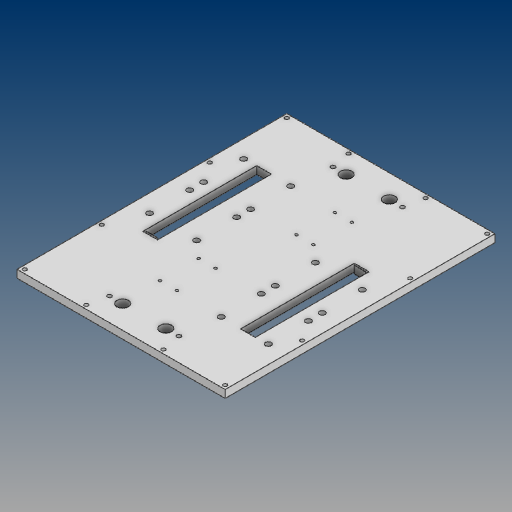
# Autodesk Inventor part: 06_Tam_de_01
Saved by Autodesk Inventor 2021 (Build 250183000, 183)
## iProperties
Created: 2024-03-25
Part Number: 06_Tam_de_01
Material: Generic
Document SubType Name: Modeling
Designer: Admin
Density: 1 g/cm^3
Appearance: Default
Author: Admin
Autodesk Inventor part; units mm, degrees
ref_plane "YZ Plane" through (0, 0, 0) normal (1, 0, 0) x (0, 1, 0)
ref_plane "XZ Plane" through (0, 0, 0) normal (0, 1, 0) x (-1, 0, 0)
ref_plane "XY Plane" through (0, 0, 0) normal (0, 0, 1) x (1, 0, 0)
sketch "Sketch1" plane through (0, 0, 0) normal (0, 1, 0) x (-1, 0, 0)
  line L0 (-135, 175) -> (135, 175)
  line L1 (135, 175) -> (135, -175)
  line L2 (135, -175) -> (-135, -175)
  line L3 (-135, -175) -> (-135, 175)
  line L4 (-135, 175) -> (135, -175) construction
  line L5 (135, 175) -> (-135, -175) construction
  point P0 (0, 0)
  dimension "d0" = 350
  dimension "d1" = 270
  constraints: 12 end point, 2 midpoint, 2 parallel, 1 horizontal, 1 perpendicular
  measures "d0" distance of L0.end L1.end
  measures "d1" distance of L1.end L2.end
extrude "Extrusion1" add sketch "Sketch1" along normal blind 10
sketch "Sketch2" plane through (0, 0, 0) normal (0, -1, 0) x (1, 0, 0)
  line L0 (135, -175) -> (-135, -175) projected
  line L1 (135, 175) -> (135, -175) projected
  line L2 (-135, 175) -> (135, 175) projected
  line L3 (-135, -175) -> (-135, 175) projected
  line L4 (130, -170) -> (-130, -170)
  line L5 (-130, -170) -> (-130, 170)
  line L6 (-130, 170) -> (130, 170)
  line L7 (130, 170) -> (130, -170)
  point P0 (0, 0)
  point P1 (50, 170)
  point P2 (130, 70)
  point P3 (130, -70)
  point P4 (50, -170)
  dimension "d4" = 5
  dimension "d5" = 80
  dimension "d6" = 100
  dimension "d7" = 100
  dimension "d8" = 80
  constraints: 8 end point, 4 point on line, 1 coincident, 3 other
  measures "d4" distance between parallel lines of L1 L7
  measures "d5" distance of L6.end point (50, 170)
  measures "d6" distance of point (130, 70) L6.end
  measures "d7" distance from line of L4 point (130, -70)
  measures "d8" distance from line of L7 point (50, -170)
hole "Hole1" at (130, 0, 170) at (50, 0, 170) at (130, 0, 70) at (130, 0, -170) at (130, 0, -70) at (50, 0, -170) direction (0, 1, 0) diameter 5 end through all
mirror "Mirror1" about plane through (0, 0, 0) normal (1, 0, 0) of "Hole1"
sketch "Sketch3" plane through (0, 10, 0) normal (0, 1, 0) x (1, 0, 0)
  line L0 (-79, 80) -> (-79, 60) projected
  line L1 (-79, 10) -> (-79, -10) projected
  line L2 (-94, -5) -> (-94, 5) projected
  line L3 (-94, 65) -> (-94, 75) projected
  spline S0 degree 3 poles (-79, -48.5854) (-84, -48.5653) (-89, -48.4297) (-94, -48.1798) knots -0.119309 -0.119309 -0.119309 -0.119309 0 0 0 0 projected
  spline S1 degree 3 poles (-79, 95.3639) (-84, 95.4408) (-89, 95.2867) (-94, 94.9058) knots -0.233196 -0.233196 -0.233196 -0.233196 0 0 0 0 projected
  line L4 (-79, -48.5854) -> (-94, -48.5854)
  line L5 (-94, -48.5854) -> (-94, 94.9058)
  line L6 (-94, 94.9058) -> (-79, 94.9058)
  line L7 (-79, 94.9058) -> (-79, -48.5854)
  line L8 (-77, -50.5854) -> (-96, -50.5854)
  line L9 (-96, -50.5854) -> (-96, 96.9058)
  line L10 (-96, 96.9058) -> (-77, 96.9058)
  line L11 (-77, 96.9058) -> (-77, -50.5854)
  point P0 (0, 0)
  dimension "d18" = 2
  constraints: 16 end point, 4 parallel, 2 perpendicular, 1 horizontal, 3 other
  measures "d18" distance between parallel lines of L7 L11
extrude "Extrusion2" cut sketch "Sketch3" against normal through all contours L0 L7 L1 S0 L5 L2 L3 L6 | L8 L9 L10 L11
pattern_circular "Circular Pattern1" count 2 over 360 about axis through (0, -10, 0) along (0, 1, 0) of "Extrusion2"
sketch "Sketch4" plane through (0, 10, 0) normal (0, 1, 0) x (1, 0, 0)
  circle A0 centre (-112, 96) radius 4 projected
  circle A1 centre (-51, 96) radius 4 projected
  circle A2 centre (-112, 44) radius 4 projected
  circle A3 centre (-51, 44) radius 4 projected
  circle A4 centre (-112, 26) radius 4 projected
  circle A5 centre (-51, 26) radius 4 projected
  circle A6 centre (-112, -26) radius 4 projected
  circle A7 centre (-51, -26) radius 4 projected
  circle A8 centre (51, 26) radius 4 projected
  circle A9 centre (112, 26) radius 4 projected
  circle A10 centre (112, -26) radius 4 projected
  circle A11 centre (51, -26) radius 4 projected
  circle A12 centre (51, -44) radius 4 projected
  circle A13 centre (51, -96) radius 4 projected
  circle A14 centre (112, -96) radius 4 projected
  circle A15 centre (112, -44) radius 4 projected
  circle A16 centre (-7.4604, -95) radius 1.75 projected
  circle A17 centre (-29.4604, -95) radius 1.75 projected
  circle A18 centre (-7.4604, -45) radius 1.75 projected
  circle A19 centre (-29.4604, -45) radius 1.75 projected
  circle A20 centre (29.4604, 95) radius 1.75 projected
  circle A21 centre (7.4604, 95) radius 1.75 projected
  circle A22 centre (7.4604, 45) radius 1.75 projected
  circle A23 centre (29.4604, 45) radius 1.75 projected
  circle A24 centre (-29.4604, -45) radius 2.25
  circle A25 centre (-7.4604, -45) radius 2.25
  circle A26 centre (-7.4604, -95) radius 2.25
  circle A27 centre (-29.4604, -95) radius 2.25
  circle A28 centre (7.4604, 45) radius 2.25
  circle A29 centre (29.4604, 45) radius 2.25
  circle A30 centre (29.4604, 95) radius 2.25
  circle A31 centre (7.4604, 95) radius 2.25
  point P0 (0, 0)
  dimension "d22" = 0.5
  dimension "d23" = 0.5
  constraints: 8 centre point, 6 equal radius, 1 coincident
  measures "d22" radial gap between concentric circles of A19 A24
  measures "d23" radial gap between concentric circles of A22 A28
hole "Hole2" at (-51, 10, -26) at (-112, 10, 26) at (-112, 10, -26) at (-112, 10, -44) at (-51, 10, 26) at (-51, 10, -96) at (-112, 10, -96) at (-51, 10, -44) at (51, 10, 26) at (51, 10, -26) at (112, 10, -26) at (112, 10, 26) at (112, 10, 44) at (112, 10, 96) at (51, 10, 96) at (51, 10, 44) direction (0, -1, 0) diameter 7.5 end through all
hole "Hole3" at (-7.4604, 10, 95) at (-29.4604, 10, 95) at (-29.4604, 10, 45) at (-7.4604, 10, 45) at (29.4604, 10, -45) at (7.4604, 10, -45) at (29.4604, 10, -95) at (7.4604, 10, -95) direction (0, -1, 0) diameter 3.5 end through all
sketch "Sketch5" plane through (0, 0, 0) normal (0, -1, 0) x (1, 0, 0)
  circle A0 centre (29.4604, -95) radius 1.75 projected
  circle A1 centre (29.4604, -45) radius 1.75 projected
  circle A2 centre (-29.4604, 45) radius 1.75 projected
  circle A3 centre (-7.4604, 95) radius 1.75 projected
  circle A4 centre (-29.4604, 95) radius 1.75 projected
  circle A5 centre (-7.4604, 45) radius 1.75 projected
  circle A6 centre (7.4604, -45) radius 1.75 projected
  circle A7 centre (7.4604, -95) radius 1.75 projected
  circle A8 centre (51, 96) radius 3.75 projected
  circle A9 centre (112, 44) radius 3.75 projected
  circle A10 centre (112, -26) radius 3.75 projected
  circle A11 centre (51, 26) radius 3.75 projected
  circle A12 centre (-112, -96) radius 3.75 projected
  circle A13 centre (-51, 26) radius 3.75 projected
  circle A14 centre (-112, -26) radius 3.75 projected
  circle A15 centre (-51, -26) radius 3.75 projected
  circle A16 centre (-112, 26) radius 3.75 projected
  circle A17 centre (-112, -44) radius 3.75 projected
  circle A18 centre (-51, -96) radius 3.75 projected
  circle A19 centre (-51, -44) radius 3.75 projected
  circle A20 centre (51, -26) radius 3.75 projected
  circle A21 centre (112, 26) radius 3.75 projected
  circle A22 centre (112, 96) radius 3.75 projected
  circle A23 centre (51, 44) radius 3.75 projected
  line L0 (-96, -96.9058) -> (-96, 50.5854) projected
  line L1 (-96, 50.5854) -> (-77, 50.5854) projected
  line L2 (-77, 50.5854) -> (-77, -96.9058) projected
  line L3 (-77, -96.9058) -> (-96, -96.9058) projected
  circle A24 centre (-130, -70) radius 2.5 projected
  circle A25 centre (-50, -170) radius 2.5 projected
  circle A26 centre (-130, -170) radius 2.5 projected
  circle A27 centre (-50, 170) radius 2.5 projected
  circle A28 centre (-130, 170) radius 2.5 projected
  circle A29 centre (-130, 70) radius 2.5 projected
  circle A30 centre (130, -70) radius 2.5 projected
  circle A31 centre (130, 70) radius 2.5 projected
  circle A32 centre (130, 170) radius 2.5 projected
  circle A33 centre (50, 170) radius 2.5 projected
  circle A34 centre (130, -170) radius 2.5 projected
  circle A35 centre (50, -170) radius 2.5 projected
  line L4 (135, -175) -> (-135, -175) projected
  line L5 (135, 175) -> (135, -175) projected
  line L6 (-135, 175) -> (135, 175) projected
  line L7 (-135, -175) -> (-135, 175) projected
  line L8 (77, -50.5854) -> (77, 96.9058) projected
  line L9 (77, 96.9058) -> (96, 96.9058) projected
  line L10 (96, 96.9058) -> (96, -50.5854) projected
  line L11 (96, -50.5854) -> (77, -50.5854) projected
  line L12 (-135, 175) -> (135, 175) projected
  line L13 (0, 175) -> (0, 145)
  line L14 (-28, 145) -> (28, 145)
  point P0 (0, 0)
  dimension "d38" = 56
  dimension "d39" = 30
  constraints: 4 end point, 2 midpoint, 1 horizontal, 1 symmetric about line, 1 vertical
  measures "d38" distance of L14.start L14.end
  measures "d39" distance between parallel lines of L6 L14
hole "Hole4" at (-28, 0, 145) at (28, 0, 145) direction (0, 1, 0) diameter 15 end through all
sketch "Sketch6" plane through (0, 0, 0) normal (0, -1, 0) x (1, 0, 0)
  circle A0 centre (-28, 145) radius 7.5 projected
  circle A1 centre (28, 145) radius 7.5 projected
  circle A2 centre (29.4604, -95) radius 1.75 projected
  circle A3 centre (29.4604, -45) radius 1.75 projected
  circle A4 centre (-29.4604, 45) radius 1.75 projected
  circle A5 centre (-7.4604, 95) radius 1.75 projected
  circle A6 centre (-29.4604, 95) radius 1.75 projected
  circle A7 centre (-7.4604, 45) radius 1.75 projected
  circle A8 centre (7.4604, -45) radius 1.75 projected
  circle A9 centre (7.4604, -95) radius 1.75 projected
  circle A10 centre (51, 96) radius 3.75 projected
  circle A11 centre (112, 44) radius 3.75 projected
  circle A12 centre (112, -26) radius 3.75 projected
  circle A13 centre (51, 26) radius 3.75 projected
  circle A14 centre (-112, -96) radius 3.75 projected
  circle A15 centre (-51, 26) radius 3.75 projected
  circle A16 centre (-112, -26) radius 3.75 projected
  circle A17 centre (-51, -26) radius 3.75 projected
  circle A18 centre (-112, 26) radius 3.75 projected
  circle A19 centre (-112, -44) radius 3.75 projected
  circle A20 centre (-51, -96) radius 3.75 projected
  circle A21 centre (-51, -44) radius 3.75 projected
  circle A22 centre (51, -26) radius 3.75 projected
  circle A23 centre (112, 26) radius 3.75 projected
  circle A24 centre (112, 96) radius 3.75 projected
  circle A25 centre (51, 44) radius 3.75 projected
  line L0 (-96, -96.9058) -> (-96, 50.5854) projected
  line L1 (-96, 50.5854) -> (-77, 50.5854) projected
  line L2 (-77, 50.5854) -> (-77, -96.9058) projected
  line L3 (-77, -96.9058) -> (-96, -96.9058) projected
  circle A26 centre (-130, -70) radius 2.5 projected
  circle A27 centre (-50, -170) radius 2.5 projected
  circle A28 centre (-130, -170) radius 2.5 projected
  circle A29 centre (-50, 170) radius 2.5 projected
  circle A30 centre (-130, 170) radius 2.5 projected
  circle A31 centre (-130, 70) radius 2.5 projected
  circle A32 centre (130, -70) radius 2.5 projected
  circle A33 centre (130, 70) radius 2.5 projected
  circle A34 centre (130, 170) radius 2.5 projected
  circle A35 centre (50, 170) radius 2.5 projected
  circle A36 centre (130, -170) radius 2.5 projected
  circle A37 centre (50, -170) radius 2.5 projected
  line L4 (135, -175) -> (-135, -175) projected
  line L5 (135, 175) -> (135, -175) projected
  line L6 (-135, 175) -> (135, 175) projected
  line L7 (-135, -175) -> (-135, 175) projected
  line L8 (77, -50.5854) -> (77, 96.9058) projected
  line L9 (77, 96.9058) -> (96, 96.9058) projected
  line L10 (96, 96.9058) -> (96, -50.5854) projected
  line L11 (96, -50.5854) -> (77, -50.5854) projected
  circle A38 centre (28, -145) radius 2.7 projected
  circle A39 centre (-28, -145) radius 2.067 projected
  line L12 (45, -145) -> (-45, -145)
  line L13 (135, -175) -> (-135, -175) projected
  line L14 (0, -175) -> (0, -137.6491)
  point P0 (0, 0)
  dimension "d47" = 90
  constraints: 4 end point, 1 horizontal, 1 midpoint, 1 perpendicular, 1 point on line, 1 symmetric about line
  measures "d47" distance of L12.start L12.end
hole "Hole5" at (-45, 0, -145) at (45, 0, -145) direction (0, 1, 0) diameter 5.5 end through all
mirror "Mirror2" about plane through (0, 0, 0) normal (0, 0, 1) of "Hole4", "Hole5"
body "Solid1"
